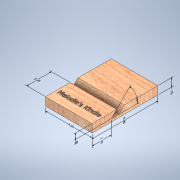
# Autodesk Inventor part: kindleStand
Saved by Autodesk Inventor 2020.2 (Build 242310000, 310)
## iProperties
Created: 2020-01-24
Part Number: kindleStand
Material: Wood (Birch)
Document SubType Name: Modeling
Designer: steele
Density: 0.55 g/cm^3
Appearance: Birch - Natural Polished
Author: steele
Autodesk Inventor part; units mm, degrees
ref_plane "YZ Plane" through (0, 0, 0) normal (1, 0, 0) x (0, 1, 0)
ref_plane "XZ Plane" through (0, 0, 0) normal (0, 1, 0) x (-1, 0, 0)
ref_plane "XY Plane" through (0, 0, 0) normal (0, 0, 1) x (1, 0, 0)
sketch "Sketch2" plane through (0, 0, 0) normal (0, 1, 0) x (-1, 0, 0)
  line L0 (53.975, 76.2) -> (-53.975, 76.2)
  line L1 (-53.975, 76.2) -> (-53.975, -76.2)
  line L2 (-53.975, -76.2) -> (53.975, -76.2)
  line L3 (53.975, -76.2) -> (53.975, 76.2)
  line L4 (53.975, 76.2) -> (-53.975, -76.2) construction
  line L5 (-53.975, 76.2) -> (53.975, -76.2) construction
  point P0 (0, 0)
  dimension "d0" = 107.95
  dimension "d1" = 152.4
  constraints: 12 end point, 2 midpoint, 2 parallel, 1 horizontal, 1 perpendicular
  measures "d0" distance of L0.start L0.end
  measures "d1" distance of L1.end L0.end
extrude "Extrusion1" add sketch "Sketch2" along normal blind 19.05
sketch "Sketch4" plane through (53.975, 0, 76.2) normal (1, 0, 0) x (0, 0, -1)
  line L0 (0, 19.05) -> (152.4, 19.05) projected
  line L1 (75.1105, 19.05) -> (62.4105, 6.35)
  line L2 (62.4105, 6.35) -> (44.45, 6.35)
  line L3 (44.45, 6.35) -> (57.15, 19.05)
  line L4 (75.1105, 19.05) -> (57.15, 19.05)
  line L5 (0, 0) -> (0, 19.05) projected
  point P0 (76.2, 0)
  point P1 (73.5162, 12.7)
  dimension "d27" = 12.7
  dimension "d28" = 44.45
  dimension "d29" = 45
  dimension "d46" = 12.7
  constraints: 8 end point, 2 parallel, 1 horizontal, 3 other
  measures "d28" distance from line of L5 L2.end
  measures "d29" angle of L3 L2
  measures "d46" distance between parallel lines of L1 L3
extrude "Extrusion3" cut sketch "Sketch4" against normal through all
sketch "Sketch6" plane through (0, 19.05, 0) normal (0, 1, 0) x (1, 0, 0)
  line L0 (-53.975, -19.05) -> (-53.975, -76.2) construction
  line L1 (-53.975, -50.8) -> (53.975, -50.8) construction
  line L2 (53.975, -76.2) -> (53.975, -19.05) construction
  line L3 (-53.975, -76.2) -> (53.975, -76.2) construction
  line L4 (-39.3515, -55.88) -> (-40.7018, -55.88)
  line L5 (-40.7018, -55.88) -> (-40.7018, -47.1279)
  line L6 (-40.7018, -47.1279) -> (-43.3529, -53.0806)
  line L7 (-43.3529, -53.0806) -> (-44.1762, -53.0806)
  line L8 (-44.1762, -53.0806) -> (-46.8027, -47.1279)
  line L9 (-46.8027, -47.1279) -> (-46.8027, -55.88)
  line L10 (-46.8027, -55.88) -> (-48.0624, -55.88)
  line L11 (-48.0624, -55.88) -> (-48.0624, -45.72)
  line L12 (-48.0624, -45.72) -> (-46.2181, -45.72)
  line L13 (-46.2181, -45.72) -> (-43.6822, -51.3763)
  line L14 (-43.6822, -51.3763) -> (-41.2287, -45.72)
  line L15 (-41.2287, -45.72) -> (-39.3515, -45.72)
  line L16 (-39.3515, -45.72) -> (-39.3515, -55.88)
  spline S0 degree 2 poles (-34.0821, -56.0529) (-35.9099, -56.0529) (-37.9189, -54.0028) (-37.9189, -52.1091) knots 0 0 0 1 2 2 2
  spline S1 degree 2 poles (-37.9189, -52.1091) (-37.9189, -50.2484) (-35.9676, -48.0418) (-34.395, -48.0418) knots 0 0 0 1 2 2 2
  spline S2 degree 2 poles (-34.395, -48.0418) (-33.6869, -48.0418) (-32.5919, -48.4535) (-32.1884, -48.8899) knots 0 0 0 1 2 2 2
  spline S3 degree 2 poles (-32.1884, -48.8899) (-31.7768, -49.3262) (-31.3404, -50.5859) (-31.3404, -51.4998) knots 0 0 0 1 2 2 2
  line L17 (-31.3404, -51.4998) -> (-31.3404, -52.1997)
  line L18 (-31.3404, -52.1997) -> (-36.618, -52.1997)
  spline S4 degree 2 poles (-36.618, -52.1997) (-36.618, -53.5253) (-35.2842, -54.9332) (-34.0986, -54.9332) knots 0 0 0 1 2 2 2
  spline S5 degree 2 poles (-34.0986, -54.9332) (-33.6787, -54.9332) (-32.8636, -54.7438) (-32.5342, -54.5956) knots 0 0 0 1 2 2 2
  spline S6 degree 2 poles (-32.5342, -54.5956) (-32.1884, -54.4309) (-31.7109, -54.1428) (-31.5545, -54.011) knots 0 0 0 1 2 2 2
  line L19 (-31.5545, -54.011) -> (-31.4804, -54.011)
  line L20 (-31.4804, -54.011) -> (-31.4804, -55.4107)
  spline S7 degree 2 poles (-31.4804, -55.4107) (-31.7027, -55.5013) (-32.3778, -55.7647) (-32.6413, -55.8388) knots 0 0 0 1 2 2 2
  spline S8 degree 2 poles (-32.6413, -55.8388) (-33.0118, -55.9459) (-33.621, -56.0529) (-34.0821, -56.0529) knots 0 0 0 1 2 2 2
  spline S9 degree 2 poles (-32.5919, -51.2199) (-32.6083, -50.7012) (-32.8224, -49.9437) (-33.0282, -49.6885) knots 0 0 0 1 2 2 2
  spline S10 degree 2 poles (-33.0282, -49.6885) (-33.2505, -49.4003) (-33.9504, -49.0957) (-34.4691, -49.0957) knots 0 0 0 1 2 2 2
  spline S11 degree 2 poles (-34.4691, -49.0957) (-34.9795, -49.0957) (-35.6959, -49.4003) (-35.9923, -49.6967) knots 0 0 0 1 2 2 2
  spline S12 degree 2 poles (-35.9923, -49.6967) (-36.2804, -50.0014) (-36.5768, -50.7341) (-36.618, -51.2199) knots 0 0 0 1 2 2 2
  line L21 (-36.618, -51.2199) -> (-32.5919, -51.2199)
  line L22 (-28.7304, -55.88) -> (-30.0148, -55.88)
  line L23 (-30.0148, -55.88) -> (-30.0148, -45.2672)
  line L24 (-30.0148, -45.2672) -> (-28.7304, -45.2672)
  line L25 (-28.7304, -45.2672) -> (-28.7304, -55.88)
  spline S13 degree 2 poles (-20.5794, -52.0679) (-20.5794, -53.9946) (-22.4319, -56.0941) (-23.9797, -56.0941) knots 0 0 0 1 2 2 2
  spline S14 degree 2 poles (-23.9797, -56.0941) (-25.5688, -56.0941) (-27.3884, -53.9287) (-27.3884, -52.0679) knots 0 0 0 1 2 2 2
  spline S15 degree 2 poles (-27.3884, -52.0679) (-27.3884, -50.1578) (-25.5112, -48.0418) (-23.9797, -48.0418) knots 0 0 0 1 2 2 2
  spline S16 degree 2 poles (-23.9797, -48.0418) (-22.4319, -48.0418) (-20.5794, -50.1496) (-20.5794, -52.0679) knots 0 0 0 1 2 2 2
  spline S17 degree 2 poles (-21.9049, -52.0679) (-21.9049, -50.5859) (-22.9835, -49.1451) (-23.9797, -49.1451) knots 0 0 0 1 2 2 2
  spline S18 degree 2 poles (-23.9797, -49.1451) (-24.976, -49.1451) (-26.0628, -50.5859) (-26.0628, -52.0679) knots 0 0 0 1 2 2 2
  spline S19 degree 2 poles (-26.0628, -52.0679) (-26.0628, -53.5088) (-24.976, -54.9908) (-23.9797, -54.9908) knots 0 0 0 1 2 2 2
  spline S20 degree 2 poles (-23.9797, -54.9908) (-22.9917, -54.9908) (-21.9049, -53.5335) (-21.9049, -52.0679) knots 0 0 0 1 2 2 2
  line L26 (-13.3998, -55.88) -> (-14.6842, -55.88)
  line L27 (-14.6842, -55.88) -> (-14.6842, -55.1061)
  spline S21 degree 2 poles (-14.6842, -55.1061) (-14.9806, -55.3531) (-15.417, -55.6824) (-15.7134, -55.8224) knots 0 0 0 1 2 2 2
  spline S22 degree 2 poles (-15.7134, -55.8224) (-15.9851, -55.9541) (-16.5697, -56.0941) (-16.9567, -56.0941) knots 0 0 0 1 2 2 2
  spline S23 degree 2 poles (-16.9567, -56.0941) (-17.5824, -56.0941) (-18.6363, -55.5754) (-19.0068, -55.0731) knots 0 0 0 1 2 2 2
  spline S24 degree 2 poles (-19.0068, -55.0731) (-19.3773, -54.5709) (-19.7889, -53.0889) (-19.7889, -52.1256) knots 0 0 0 1 2 2 2
  spline S25 degree 2 poles (-19.7889, -52.1256) (-19.7889, -51.1211) (-19.2702, -49.6556) (-18.8174, -49.1039) knots 0 0 0 1 2 2 2
  spline S26 degree 2 poles (-18.8174, -49.1039) (-18.3975, -48.6099) (-17.2201, -48.0418) (-16.5697, -48.0418) knots 0 0 0 1 2 2 2
  spline S27 degree 2 poles (-16.5697, -48.0418) (-16.0016, -48.0418) (-15.1535, -48.2971) (-14.6842, -48.5605) knots 0 0 0 1 2 2 2
  line L28 (-14.6842, -48.5605) -> (-14.6842, -45.2672)
  line L29 (-14.6842, -45.2672) -> (-13.3998, -45.2672)
  line L30 (-13.3998, -45.2672) -> (-13.3998, -55.88)
  line L31 (-14.6842, -54.0275) -> (-14.6842, -49.6226)
  spline S28 degree 2 poles (-14.6842, -49.6226) (-15.1618, -49.3921) (-15.9193, -49.2192) (-16.3556, -49.2192) knots 0 0 0 1 2 2 2
  spline S29 degree 2 poles (-16.3556, -49.2192) (-17.3436, -49.2192) (-18.4634, -50.7012) (-18.4634, -52.1009) knots 0 0 0 1 2 2 2
  spline S30 degree 2 poles (-18.4634, -52.1009) (-18.4634, -53.4512) (-17.6071, -54.8755) (-16.6603, -54.8755) knots 0 0 0 1 2 2 2
  spline S31 degree 2 poles (-16.6603, -54.8755) (-16.158, -54.8755) (-15.1371, -54.4145) (-14.6842, -54.0275) knots 0 0 0 1 2 2 2
  line L32 (-10.23, -55.88) -> (-11.5144, -55.88)
  line L33 (-11.5144, -55.88) -> (-11.5144, -48.2559)
  line L34 (-11.5144, -48.2559) -> (-10.23, -48.2559)
  line L35 (-10.23, -48.2559) -> (-10.23, -55.88)
  line L36 (-10.1394, -46.9879) -> (-11.5967, -46.9879)
  line L37 (-11.5967, -46.9879) -> (-11.5967, -45.6541)
  line L38 (-11.5967, -45.6541) -> (-10.1394, -45.6541)
  line L39 (-10.1394, -45.6541) -> (-10.1394, -46.9879)
  spline S32 degree 2 poles (-5.0347, -56.0529) (-6.8625, -56.0529) (-8.8715, -54.0028) (-8.8715, -52.1091) knots 0 0 0 1 2 2 2
  spline S33 degree 2 poles (-8.8715, -52.1091) (-8.8715, -50.2484) (-6.9202, -48.0418) (-5.3476, -48.0418) knots 0 0 0 1 2 2 2
  spline S34 degree 2 poles (-5.3476, -48.0418) (-4.6395, -48.0418) (-3.5445, -48.4535) (-3.141, -48.8899) knots 0 0 0 1 2 2 2
  spline S35 degree 2 poles (-3.141, -48.8899) (-2.7294, -49.3262) (-2.293, -50.5859) (-2.293, -51.4998) knots 0 0 0 1 2 2 2
  line L40 (-2.293, -51.4998) -> (-2.293, -52.1997)
  line L41 (-2.293, -52.1997) -> (-7.5706, -52.1997)
  spline S36 degree 2 poles (-7.5706, -52.1997) (-7.5706, -53.5253) (-6.2368, -54.9332) (-5.0512, -54.9332) knots 0 0 0 1 2 2 2
  spline S37 degree 2 poles (-5.0512, -54.9332) (-4.6313, -54.9332) (-3.8162, -54.7438) (-3.4868, -54.5956) knots 0 0 0 1 2 2 2
  spline S38 degree 2 poles (-3.4868, -54.5956) (-3.141, -54.4309) (-2.6635, -54.1428) (-2.5071, -54.011) knots 0 0 0 1 2 2 2
  line L42 (-2.5071, -54.011) -> (-2.433, -54.011)
  line L43 (-2.433, -54.011) -> (-2.433, -55.4107)
  spline S39 degree 2 poles (-2.433, -55.4107) (-2.6553, -55.5013) (-3.3304, -55.7647) (-3.5939, -55.8388) knots 0 0 0 1 2 2 2
  spline S40 degree 2 poles (-3.5939, -55.8388) (-3.9644, -55.9459) (-4.5736, -56.0529) (-5.0347, -56.0529) knots 0 0 0 1 2 2 2
  spline S41 degree 2 poles (-3.5445, -51.2199) (-3.5609, -50.7012) (-3.775, -49.9437) (-3.9808, -49.6885) knots 0 0 0 1 2 2 2
  spline S42 degree 2 poles (-3.9808, -49.6885) (-4.2031, -49.4003) (-4.903, -49.0957) (-5.4217, -49.0957) knots 0 0 0 1 2 2 2
  spline S43 degree 2 poles (-5.4217, -49.0957) (-5.9322, -49.0957) (-6.6485, -49.4003) (-6.9449, -49.6967) knots 0 0 0 1 2 2 2
  spline S44 degree 2 poles (-6.9449, -49.6967) (-7.233, -50.0014) (-7.5294, -50.7341) (-7.5706, -51.2199) knots 0 0 0 1 2 2 2
  line L44 (-7.5706, -51.2199) -> (-3.5445, -51.2199)
  line L45 (0.3088, -45.2672) -> (0.0124, -49.2192)
  line L46 (0.0124, -49.2192) -> (-0.9098, -49.2192)
  line L47 (-0.9098, -49.2192) -> (-1.2062, -45.2672)
  line L48 (-1.2062, -45.2672) -> (0.3088, -45.2672)
  spline S45 degree 2 poles (4.0138, -56.0611) (3.2481, -56.0611) (1.9225, -55.6495) (1.4861, -55.4189) knots 0 0 0 1 2 2 2
  line L49 (1.4861, -55.4189) -> (1.4861, -53.9781)
  line L50 (1.4861, -53.9781) -> (1.552, -53.9781)
  spline S46 degree 2 poles (1.552, -53.9781) (1.7167, -54.1098) (2.1613, -54.4227) (2.5318, -54.5956) knots 0 0 0 1 2 2 2
  spline S47 degree 2 poles (2.5318, -54.5956) (2.8529, -54.752) (3.6433, -54.9826) (4.0632, -54.9826) knots 0 0 0 1 2 2 2
  spline S48 degree 2 poles (4.0632, -54.9826) (4.3678, -54.9826) (5.0677, -54.8426) (5.2323, -54.7273) knots 0 0 0 1 2 2 2
  spline S49 degree 2 poles (5.2323, -54.7273) (5.4711, -54.5709) (5.6852, -54.2169) (5.6852, -53.8546) knots 0 0 0 1 2 2 2
  spline S50 degree 2 poles (5.6852, -53.8546) (5.6852, -53.4018) (5.1912, -52.9324) (4.5572, -52.776) knots 0 0 0 1 2 2 2
  spline S51 degree 2 poles (4.5572, -52.776) (4.3102, -52.7184) (3.5198, -52.5537) (3.1822, -52.4631) knots 0 0 0 1 2 2 2
  spline S52 degree 2 poles (3.1822, -52.4631) (2.3095, -52.2079) (1.5191, -51.154) (1.5191, -50.4048) knots 0 0 0 1 2 2 2
  spline S53 degree 2 poles (1.5191, -50.4048) (1.5191, -49.3674) (3.0752, -48.0747) (4.3596, -48.0747) knots 0 0 0 1 2 2 2
  spline S54 degree 2 poles (4.3596, -48.0747) (4.9936, -48.0747) (6.278, -48.3876) (6.7143, -48.6264) knots 0 0 0 1 2 2 2
  line L51 (6.7143, -48.6264) -> (6.7143, -50.0014)
  line L52 (6.7143, -50.0014) -> (6.6485, -50.0014)
  spline S55 degree 2 poles (6.6485, -50.0014) (6.1545, -49.6062) (4.9524, -49.1533) (4.3349, -49.1533) knots 0 0 0 1 2 2 2
  spline S56 degree 2 poles (4.3349, -49.1533) (3.7009, -49.1533) (2.8282, -49.6885) (2.8282, -50.2237) knots 0 0 0 1 2 2 2
  spline S57 degree 2 poles (2.8282, -50.2237) (2.8282, -50.7094) (3.3469, -51.1787) (3.9232, -51.3269) knots 0 0 0 1 2 2 2
  spline S58 degree 2 poles (3.9232, -51.3269) (4.2031, -51.401) (4.9112, -51.5492) (5.2982, -51.6398) knots 0 0 0 1 2 2 2
  spline S59 degree 2 poles (5.2982, -51.6398) (6.138, -51.8539) (6.9943, -52.8336) (6.9943, -53.6817) knots 0 0 0 1 2 2 2
  spline S60 degree 2 poles (6.9943, -53.6817) (6.9943, -54.1757) (6.6073, -55.0484) (6.2286, -55.3695) knots 0 0 0 1 2 2 2
  spline S61 degree 2 poles (6.2286, -55.3695) (5.8251, -55.7071) (4.7959, -56.0611) (4.0138, -56.0611) knots 0 0 0 1 2 2 2
  line L53 (20.0606, -55.88) -> (18.3069, -55.88)
  line L54 (18.3069, -55.88) -> (14.5937, -51.154)
  line L55 (14.5937, -51.154) -> (14.0009, -51.8209)
  line L56 (14.0009, -51.8209) -> (14.0009, -55.88)
  line L57 (14.0009, -55.88) -> (12.6506, -55.88)
  line L58 (12.6506, -55.88) -> (12.6506, -45.72)
  line L59 (12.6506, -45.72) -> (14.0009, -45.72)
  line L60 (14.0009, -45.72) -> (14.0009, -50.3883)
  line L61 (14.0009, -50.3883) -> (18.167, -45.72)
  line L62 (18.167, -45.72) -> (19.8136, -45.72)
  line L63 (19.8136, -45.72) -> (15.6064, -50.2566)
  line L64 (15.6064, -50.2566) -> (20.0606, -55.88)
  line L65 (22.0778, -55.88) -> (20.7934, -55.88)
  line L66 (20.7934, -55.88) -> (20.7934, -48.2559)
  line L67 (20.7934, -48.2559) -> (22.0778, -48.2559)
  line L68 (22.0778, -48.2559) -> (22.0778, -55.88)
  line L69 (22.1684, -46.9879) -> (20.7111, -46.9879)
  line L70 (20.7111, -46.9879) -> (20.7111, -45.6541)
  line L71 (20.7111, -45.6541) -> (22.1684, -45.6541)
  line L72 (22.1684, -45.6541) -> (22.1684, -46.9879)
  line L73 (29.9489, -55.88) -> (28.6645, -55.88)
  line L74 (28.6645, -55.88) -> (28.6645, -51.5328)
  spline S62 degree 2 poles (28.6645, -51.5328) (28.6645, -51.0058) (28.5657, -50.1002) (28.4175, -49.8285) knots 0 0 0 1 2 2 2
  spline S63 degree 2 poles (28.4175, -49.8285) (28.2611, -49.5403) (27.7012, -49.2604) (27.2237, -49.2604) knots 0 0 0 1 2 2 2
  spline S64 degree 2 poles (27.2237, -49.2604) (26.7462, -49.2604) (25.7335, -49.7708) (25.2477, -50.1825) knots 0 0 0 1 2 2 2
  line L75 (25.2477, -50.1825) -> (25.2477, -55.88)
  line L76 (25.2477, -55.88) -> (23.9633, -55.88)
  line L77 (23.9633, -55.88) -> (23.9633, -48.2559)
  line L78 (23.9633, -48.2559) -> (25.2477, -48.2559)
  line L79 (25.2477, -48.2559) -> (25.2477, -49.1039)
  spline S65 degree 2 poles (25.2477, -49.1039) (25.824, -48.5852) (26.9355, -48.0418) (27.5613, -48.0418) knots 0 0 0 1 2 2 2
  spline S66 degree 2 poles (27.5613, -48.0418) (28.681, -48.0418) (29.9489, -49.5238) (29.9489, -50.9317) knots 0 0 0 1 2 2 2
  line L80 (29.9489, -50.9317) -> (29.9489, -55.88)
  line L81 (37.6142, -55.88) -> (36.3298, -55.88)
  line L82 (36.3298, -55.88) -> (36.3298, -55.1061)
  spline S67 degree 2 poles (36.3298, -55.1061) (36.0334, -55.3531) (35.5971, -55.6824) (35.3006, -55.8224) knots 0 0 0 1 2 2 2
  spline S68 degree 2 poles (35.3006, -55.8224) (35.0289, -55.9541) (34.4444, -56.0941) (34.0574, -56.0941) knots 0 0 0 1 2 2 2
  spline S69 degree 2 poles (34.0574, -56.0941) (33.4317, -56.0941) (32.3778, -55.5754) (32.0073, -55.0731) knots 0 0 0 1 2 2 2
  spline S70 degree 2 poles (32.0073, -55.0731) (31.6368, -54.5709) (31.2251, -53.0889) (31.2251, -52.1256) knots 0 0 0 1 2 2 2
  spline S71 degree 2 poles (31.2251, -52.1256) (31.2251, -51.1211) (31.7438, -49.6556) (32.1967, -49.1039) knots 0 0 0 1 2 2 2
  spline S72 degree 2 poles (32.1967, -49.1039) (32.6166, -48.6099) (33.7939, -48.0418) (34.4444, -48.0418) knots 0 0 0 1 2 2 2
  spline S73 degree 2 poles (34.4444, -48.0418) (35.0125, -48.0418) (35.8605, -48.2971) (36.3298, -48.5605) knots 0 0 0 1 2 2 2
  line L83 (36.3298, -48.5605) -> (36.3298, -45.2672)
  line L84 (36.3298, -45.2672) -> (37.6142, -45.2672)
  line L85 (37.6142, -45.2672) -> (37.6142, -55.88)
  line L86 (36.3298, -54.0275) -> (36.3298, -49.6226)
  spline S74 degree 2 poles (36.3298, -49.6226) (35.8523, -49.3921) (35.0948, -49.2192) (34.6584, -49.2192) knots 0 0 0 1 2 2 2
  spline S75 degree 2 poles (34.6584, -49.2192) (33.6704, -49.2192) (32.5507, -50.7012) (32.5507, -52.1009) knots 0 0 0 1 2 2 2
  spline S76 degree 2 poles (32.5507, -52.1009) (32.5507, -53.4512) (33.407, -54.8755) (34.3538, -54.8755) knots 0 0 0 1 2 2 2
  spline S77 degree 2 poles (34.3538, -54.8755) (34.856, -54.8755) (35.877, -54.4145) (36.3298, -54.0275) knots 0 0 0 1 2 2 2
  line L87 (40.7841, -55.88) -> (39.4997, -55.88)
  line L88 (39.4997, -55.88) -> (39.4997, -45.2672)
  line L89 (39.4997, -45.2672) -> (40.7841, -45.2672)
  line L90 (40.7841, -45.2672) -> (40.7841, -55.88)
  spline S78 degree 2 poles (45.9794, -56.0529) (44.1515, -56.0529) (42.1426, -54.0028) (42.1426, -52.1091) knots 0 0 0 1 2 2 2
  spline S79 degree 2 poles (42.1426, -52.1091) (42.1426, -50.2484) (44.0939, -48.0418) (45.6665, -48.0418) knots 0 0 0 1 2 2 2
  spline S80 degree 2 poles (45.6665, -48.0418) (46.3746, -48.0418) (47.4696, -48.4535) (47.873, -48.8899) knots 0 0 0 1 2 2 2
  spline S81 degree 2 poles (47.873, -48.8899) (48.2847, -49.3262) (48.7211, -50.5859) (48.7211, -51.4998) knots 0 0 0 1 2 2 2
  line L91 (48.7211, -51.4998) -> (48.7211, -52.1997)
  line L92 (48.7211, -52.1997) -> (43.4435, -52.1997)
  spline S82 degree 2 poles (43.4435, -52.1997) (43.4435, -53.5253) (44.7773, -54.9332) (45.9629, -54.9332) knots 0 0 0 1 2 2 2
  spline S83 degree 2 poles (45.9629, -54.9332) (46.3828, -54.9332) (47.1979, -54.7438) (47.5272, -54.5956) knots 0 0 0 1 2 2 2
  spline S84 degree 2 poles (47.5272, -54.5956) (47.873, -54.4309) (48.3506, -54.1428) (48.507, -54.011) knots 0 0 0 1 2 2 2
  line L93 (48.507, -54.011) -> (48.5811, -54.011)
  line L94 (48.5811, -54.011) -> (48.5811, -55.4107)
  spline S85 degree 2 poles (48.5811, -55.4107) (48.3588, -55.5013) (47.6837, -55.7647) (47.4202, -55.8388) knots 0 0 0 1 2 2 2
  spline S86 degree 2 poles (47.4202, -55.8388) (47.0497, -55.9459) (46.4404, -56.0529) (45.9794, -56.0529) knots 0 0 0 1 2 2 2
  spline S87 degree 2 poles (47.4696, -51.2199) (47.4531, -50.7012) (47.2391, -49.9437) (47.0332, -49.6885) knots 0 0 0 1 2 2 2
  spline S88 degree 2 poles (47.0332, -49.6885) (46.8109, -49.4003) (46.1111, -49.0957) (45.5924, -49.0957) knots 0 0 0 1 2 2 2
  spline S89 degree 2 poles (45.5924, -49.0957) (45.0819, -49.0957) (44.3656, -49.4003) (44.0692, -49.6967) knots 0 0 0 1 2 2 2
  spline S90 degree 2 poles (44.0692, -49.6967) (43.781, -50.0014) (43.4846, -50.7341) (43.4435, -51.2199) knots 0 0 0 1 2 2 2
  line L95 (43.4435, -51.2199) -> (47.4696, -51.2199)
  point P0 (0, 0)
  dimension "d50" = 25.4
  constraints: 2 end point, 2 horizontal, 2 point on line
  measures "d50" distance between parallel lines of L1 L3
extrude "Extrusion4" cut sketch "Sketch6" against normal blind 2.54
body "Solid1"
